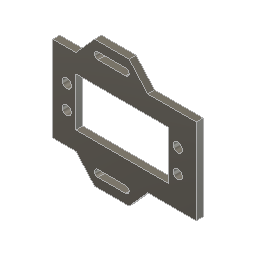
SteeringServoPlatform (Autodesk Fusion 360 design; units mm, degrees)
Autodesk Fusion 360 part; units mm, degrees
sketch "Sketch1" plane through (0, 0, 0) normal (0, 0, 1) x (1, 0, 0)
  line L0 (33.7043, 31.4724) -> (95.7043, 31.4724)
  line L1 (95.7043, 31.4724) -> (95.7043, -5.5276)
  line L2 (95.7043, -5.5276) -> (33.7043, -5.5276)
  line L3 (33.7043, -5.5276) -> (33.7043, 31.4724)
  line L4 (33.7043, 31.4724) -> (43.7043, 31.4724)
  line L5 (43.7043, 31.4724) -> (43.7043, -5.5276)
  line L6 (43.7043, -5.5276) -> (33.7043, -5.5276)
  line L7 (33.7043, -5.5276) -> (33.7043, 31.4724)
  line L8 (95.7043, 31.4724) -> (83.7043, 31.4724)
  line L9 (83.7043, 31.4724) -> (83.7043, -5.5276)
  line L10 (83.7043, -5.5276) -> (95.7043, -5.5276)
  line L11 (95.7043, -5.5276) -> (95.7043, 31.4724)
  line L12 (33.7043, -5.5276) -> (95.7282, -5.5276)
  line L13 (95.7282, -5.5276) -> (95.7282, 2.4724)
  line L14 (95.7282, 2.4724) -> (33.7043, 2.4724)
  line L15 (33.7043, 2.4724) -> (33.7043, -5.5276)
  line L16 (33.7043, 31.4724) -> (95.7282, 31.4724)
  line L17 (95.7282, 31.4724) -> (95.7282, 23.4724)
  line L18 (95.7282, 23.4724) -> (33.7043, 23.4724)
  line L19 (33.7043, 23.4724) -> (33.7043, 31.4724)
  line L20 (33.7043, 2.4724) -> (95.7282, 2.4724)
  line L21 (95.7282, 2.4724) -> (95.7282, -14.5276)
  line L22 (95.7282, -14.5276) -> (33.7043, -14.5276)
  line L23 (33.7043, -14.5276) -> (33.7043, 2.4724)
  line L24 (33.7043, 23.4724) -> (95.7282, 23.4724)
  line L25 (95.7282, 23.4724) -> (95.7282, 40.4724)
  line L26 (95.7282, 40.4724) -> (33.7043, 40.4724)
  line L27 (33.7043, 40.4724) -> (33.7043, 23.4724)
  line L28 (33.7043, -14.5276) -> (95.7282, -14.5276)
  line L29 (95.7282, -14.5276) -> (95.7282, -10.5276)
  line L30 (95.7282, -10.5276) -> (33.7043, -10.5276)
  line L31 (33.7043, -10.5276) -> (33.7043, -14.5276)
  line L32 (33.7043, 40.4724) -> (95.7282, 40.4724)
  line L33 (95.7282, 40.4724) -> (95.7282, 36.4724)
  line L34 (95.7282, 36.4724) -> (33.7043, 36.4724)
  line L35 (33.7043, 36.4724) -> (33.7043, 40.4724)
  line L36 (33.7043, 36.4724) -> (51.7043, 36.4724)
  line L37 (51.7043, 36.4724) -> (51.7043, 31.4724)
  line L38 (51.7043, 31.4724) -> (33.7043, 31.4724)
  line L39 (33.7043, 31.4724) -> (33.7043, 36.4724)
  line L40 (33.7043, -5.5276) -> (51.7043, -5.5276)
  line L41 (51.7043, -5.5276) -> (51.7043, -10.5276)
  line L42 (51.7043, -10.5276) -> (33.7043, -10.5276)
  line L43 (33.7043, -10.5276) -> (33.7043, -5.5276)
  line L44 (51.7043, 36.4724) -> (66.7043, 36.4724)
  line L45 (66.7043, 36.4724) -> (66.7043, 31.4724)
  line L46 (66.7043, 31.4724) -> (51.7043, 31.4724)
  line L47 (51.7043, 31.4724) -> (51.7043, 36.4724)
  line L48 (51.7043, -5.5276) -> (66.7043, -5.5276)
  line L49 (66.7043, -5.5276) -> (66.7043, -10.5276)
  line L50 (66.7043, -10.5276) -> (51.7043, -10.5276)
  line L51 (51.7043, -10.5276) -> (51.7043, -5.5276)
  line L52 (33.7043, -5.5276) -> (95.7282, -5.5276)
  line L53 (95.7282, -5.5276) -> (95.7282, -7.5276)
  line L54 (95.7282, -7.5276) -> (33.7043, -7.5276)
  line L55 (33.7043, -7.5276) -> (33.7043, -5.5276)
  line L56 (33.7043, 31.4724) -> (95.7282, 31.4724)
  line L57 (95.7282, 31.4724) -> (95.7282, 33.4724)
  line L58 (95.7282, 33.4724) -> (33.7043, 33.4724)
  line L59 (33.7043, 33.4724) -> (33.7043, 31.4724)
  line L60 (51.7043, -10.5276) -> (51.7043, -14.5276)
  line L61 (66.7043, -10.5276) -> (66.7043, -14.5276)
  line L62 (51.7043, 36.4724) -> (51.7043, 40.4724)
  line L63 (66.7043, 36.4724) -> (66.7043, 40.4724)
  line L64 (43.7043, 31.4724) -> (51.7043, 40.4724)
  line L65 (43.7043, -5.5276) -> (51.7043, -14.5276)
  line L66 (66.7043, 31.4724) -> (74.7043, 31.4724)
  line L67 (74.7043, 31.4724) -> (74.7043, 40.4724)
  line L68 (74.7043, 40.4724) -> (66.7043, 40.4724)
  line L69 (66.7043, 40.4724) -> (66.7043, 31.4724)
  line L70 (66.7043, 40.4724) -> (74.7043, 31.4724)
  line L71 (66.7043, -5.5276) -> (74.7043, -5.5276)
  line L72 (74.7043, -5.5276) -> (74.7043, -14.5276)
  line L73 (74.7043, -14.5276) -> (66.7043, -14.5276)
  line L74 (66.7043, -14.5276) -> (66.7043, -5.5276)
  line L75 (66.7043, -14.5276) -> (74.7043, -5.5276)
  line L76 (43.7043, 12.9724) -> (41.7043, 12.9724)
  line L77 (41.7043, 12.9724) -> (41.7043, 7.9724)
  line L78 (41.7043, 7.9724) -> (43.7043, 7.9724)
  line L79 (43.7043, 7.9724) -> (43.7043, 12.9724)
  line L80 (43.7043, 12.9724) -> (41.7043, 12.9724)
  line L81 (41.7043, 12.9724) -> (41.7043, 17.9724)
  line L82 (41.7043, 17.9724) -> (43.7043, 17.9724)
  line L83 (43.7043, 17.9724) -> (43.7043, 12.9724)
  line L84 (41.7043, 7.9697) -> (41.7043, 17.9724)
  line L85 (41.7043, 17.9724) -> (37.7043, 17.9724)
  line L86 (37.7043, 17.9724) -> (37.7043, 7.9724)
  line L87 (37.7043, 7.9724) -> (41.7043, 7.9724)
  line L88 (41.7043, 7.9724) -> (41.7043, 17.9724)
  circle A0 centre (39.7043, 17.9724) radius 2
  circle A1 centre (39.7043, 7.9724) radius 2
  line L89 (43.7043, 17.9724) -> (43.7043, 12.9724)
  line L90 (41.7043, 7.9724) -> (41.7043, 17.9724)
  line L91 (41.7043, 12.9724) -> (41.7043, 17.9724)
  line L92 (37.7043, 17.9724) -> (37.7043, 7.9724)
  line L93 (43.7043, 7.9724) -> (43.7043, 12.9724)
  line L94 (41.7043, 7.9697) -> (41.7043, 17.9724)
  circle A2 centre (39.7043, 7.9724) radius 2
  line L95 (43.7043, 12.9724) -> (41.7043, 12.9724)
  line L96 (41.7043, 12.9724) -> (41.7043, 7.9724)
  line L97 (41.7043, 17.9724) -> (37.7043, 17.9724)
  line L98 (41.7043, 7.9724) -> (43.7043, 7.9724)
  circle A3 centre (39.7043, 17.9724) radius 2
  line L99 (43.7043, 12.9724) -> (41.7043, 12.9724)
  line L100 (37.7043, 7.9724) -> (41.7043, 7.9724)
  line L101 (41.7043, 17.9724) -> (43.7043, 17.9724)
  line L102 (41.7043, 7.9697) -> (41.7043, 17.9724)
  line L103 (43.7043, 12.9724) -> (41.7043, 12.9724)
  line L104 (41.7043, 17.9724) -> (43.7043, 17.9724)
  line L105 (41.7043, 17.9724) -> (37.7043, 17.9724)
  line L106 (41.7043, 17.9724) -> (37.7043, 17.9724)
  circle A4 centre (39.7043, 17.9724) radius 2
  circle A5 centre (39.7043, 7.9724) radius 2
  line L107 (43.7043, 7.9724) -> (43.7043, 12.9724)
  line L108 (43.7043, 12.9724) -> (41.7043, 12.9724)
  line L109 (41.7043, 7.9697) -> (41.7043, 17.9724)
  circle A6 centre (39.7043, 17.9724) radius 2
  line L110 (43.7043, 12.9724) -> (41.7043, 12.9724)
  line L111 (37.7043, 7.9724) -> (41.7043, 7.9724)
  line L112 (41.7043, 7.9724) -> (43.7043, 7.9724)
  line L113 (41.7043, 17.9724) -> (43.7043, 17.9724)
  line L114 (41.7043, 7.9724) -> (41.7043, 17.9724)
  line L115 (37.7043, 17.9724) -> (37.7043, 7.9724)
  circle A7 centre (39.7043, 7.9724) radius 2
  line L116 (37.7043, 7.9724) -> (41.7043, 7.9724)
  line L117 (41.7043, 12.9724) -> (41.7043, 7.9724)
  line L118 (43.7043, 7.9724) -> (43.7043, 12.9724)
  line L119 (37.7043, 17.9724) -> (37.7043, 7.9724)
  line L120 (41.7043, 12.9724) -> (41.7043, 17.9724)
  line L121 (43.7043, 12.9724) -> (41.7043, 12.9724)
  line L122 (41.7043, 7.9724) -> (41.7043, 17.9724)
  line L123 (43.7043, 17.9724) -> (43.7043, 12.9724)
  line L124 (43.7043, 17.9724) -> (43.7043, 12.9724)
  line L125 (41.7043, 7.9724) -> (43.7043, 7.9724)
  line L126 (41.7043, 12.9724) -> (41.7043, 7.9724)
  line L127 (41.7043, 12.9724) -> (41.7043, 17.9724)
  line L128 (85.7043, 7.9724) -> (85.7043, 17.9724)
  line L129 (85.7043, 12.9724) -> (85.7043, 17.9724)
  line L130 (85.7043, 7.9697) -> (85.7043, 17.9724)
  line L131 (89.7043, 17.9724) -> (89.7043, 7.9724)
  line L132 (89.7043, 17.9724) -> (89.7043, 7.9724)
  line L133 (83.7043, 17.9724) -> (83.7043, 12.9724)
  line L134 (85.7043, 17.9724) -> (89.7043, 17.9724)
  line L135 (83.7043, 12.9724) -> (85.7043, 12.9724)
  line L136 (85.7043, 12.9724) -> (85.7043, 7.9724)
  line L137 (85.7043, 17.9724) -> (83.7043, 17.9724)
  line L138 (89.7043, 7.9724) -> (85.7043, 7.9724)
  circle A8 centre (87.7043, 17.9724) radius 2
  line L139 (83.7043, 12.9724) -> (85.7043, 12.9724)
  line L140 (85.7043, 7.9724) -> (83.7043, 7.9724)
  line L141 (83.7043, 12.9724) -> (85.7043, 12.9724)
  circle A9 centre (87.7043, 17.9724) radius 2
  line L142 (85.7043, 7.9724) -> (83.7043, 7.9724)
  line L143 (83.7043, 7.9724) -> (83.7043, 12.9724)
  circle A10 centre (87.7043, 7.9724) radius 2
  line L144 (85.7043, 7.9724) -> (83.7043, 7.9724)
  circle A11 centre (87.7043, 17.9724) radius 2
  line L145 (83.7043, 12.9724) -> (85.7043, 12.9724)
  line L146 (85.7043, 17.9724) -> (89.7043, 17.9724)
  line L147 (83.7043, 12.9724) -> (85.7043, 12.9724)
  circle A12 centre (87.7043, 17.9724) radius 2
  line L148 (85.7043, 17.9724) -> (83.7043, 17.9724)
  line L149 (85.7043, 17.9724) -> (83.7043, 17.9724)
  line L150 (85.7043, 17.9724) -> (89.7043, 17.9724)
  line L151 (85.7043, 17.9724) -> (83.7043, 17.9724)
  line L152 (85.7043, 17.9724) -> (89.7043, 17.9724)
  circle A13 centre (87.7043, 7.9724) radius 2
  line L153 (89.7043, 7.9724) -> (85.7043, 7.9724)
  line L154 (85.7043, 12.9724) -> (85.7043, 17.9724)
  line L155 (89.7043, 7.9724) -> (85.7043, 7.9724)
  line L156 (85.7043, 12.9724) -> (85.7043, 17.9724)
  line L157 (83.7043, 7.9724) -> (83.7043, 12.9724)
  line L158 (89.7043, 7.9724) -> (85.7043, 7.9724)
  circle A14 centre (87.7043, 7.9724) radius 2
  line L159 (83.7043, 17.9724) -> (83.7043, 12.9724)
  line L160 (85.7043, 7.9724) -> (85.7043, 17.9724)
  line L161 (85.7043, 12.9724) -> (85.7043, 17.9724)
  line L162 (85.7043, 7.9697) -> (85.7043, 17.9724)
  line L163 (89.7043, 17.9724) -> (89.7043, 7.9724)
  line L164 (85.7043, 7.9724) -> (85.7043, 17.9724)
  line L165 (89.7043, 17.9724) -> (89.7043, 7.9724)
  line L166 (85.7043, 7.9724) -> (85.7043, 17.9724)
  line L167 (83.7043, 17.9724) -> (83.7043, 12.9724)
  line L168 (85.7043, 7.9724) -> (83.7043, 7.9724)
  line L169 (83.7043, 12.9724) -> (85.7043, 12.9724)
  line L170 (85.7043, 12.9724) -> (85.7043, 7.9724)
  line L171 (85.7043, 12.9724) -> (85.7043, 7.9724)
  line L172 (85.7043, 12.9724) -> (85.7043, 7.9724)
  line L173 (85.7043, 7.9697) -> (85.7043, 17.9724)
  line L174 (83.7043, 17.9724) -> (83.7043, 12.9724)
  line L175 (85.7043, 7.9697) -> (85.7043, 17.9724)
  line L176 (83.7043, 7.9724) -> (83.7043, 12.9724)
  line L177 (83.7043, 12.9724) -> (85.7043, 12.9724)
  line L178 (83.7043, 12.9724) -> (85.7043, 12.9724)
  line L179 (83.7043, 7.9724) -> (83.7043, 12.9724)
  circle A15 centre (87.7043, 7.9724) radius 2
  circle A16 centre (65.2043, 34.9724) radius 1.5
  circle A17 centre (53.2043, 34.9724) radius 1.5
  circle A18 centre (53.2043, -9.0276) radius 1.5
  circle A19 centre (65.2043, -9.0276) radius 1.5
  dimension "d1" = 62
  dimension "d2" = 37
  dimension "d3" = 10
  dimension "d4" = 12
  dimension "d5" = 8
  dimension "d6" = 8
  dimension "d7" = 17
  dimension "d8" = 17
  dimension "d9" = 4
  dimension "d10" = 4
  dimension "d11" = 18
  dimension "d12" = 18
  dimension "d13" = 15
  dimension "d14" = 15
  dimension "d15" = 2
  dimension "d16" = 2
  dimension "d17" = 4
  dimension "d18" = 4
  dimension "d19" = 4
  dimension "d20" = 4
  dimension "d21" = 8
  dimension "d22" = 8
  dimension "d23" = 2
  dimension "d24" = 5
  dimension "d25" = 2
  dimension "d26" = 5
  dimension "d30" = 4
  dimension "d31" = 4
  dimension "d32" = 4
  dimension "d33" = 2
  dimension "d34" = 5
  dimension "d35" = 2
  dimension "d36" = 5
  dimension "d37" = 4
  dimension "d38" = 4
  dimension "d39" = 4
  dimension "d40" = 2
  dimension "d41" = 5
  dimension "d42" = 2
  dimension "d43" = 5
  dimension "d44" = 4
  dimension "d45" = 4
  dimension "d46" = 4
  dimension "d47" = 2
  dimension "d48" = 5
  dimension "d49" = 2
  dimension "d50" = 5
  dimension "d51" = 4
  dimension "d52" = 4
  dimension "d53" = 4
  dimension "d54" = 2
  dimension "d55" = 5
  dimension "d56" = 2
  dimension "d57" = 5
  dimension "d58" = 4
  dimension "d59" = 4
  dimension "d60" = 4
  dimension "d61" = 2
  dimension "d62" = 5
  dimension "d63" = 2
  dimension "d64" = 5
  dimension "d65" = 4
  dimension "d66" = 4
  dimension "d67" = 4
  dimension "d68" = 2
  dimension "d69" = 5
  dimension "d70" = 2
  dimension "d71" = 5
  dimension "d72" = 4
  dimension "d73" = 4
  dimension "d74" = 4
  dimension "d75" = 2
  dimension "d76" = 5
  dimension "d77" = 2
  dimension "d78" = 5
  dimension "d79" = 4
  dimension "d80" = 4
  dimension "d81" = 4
  dimension "d82" = 3
  dimension "d83" = 3
  dimension "d84" = 3
  dimension "d85" = 3
  constraint horizontal L0
  constraint vertical L1
  constraint horizontal L2
  constraint vertical L3
  constraint horizontal L4
  constraint vertical L5
  constraint horizontal L6
  constraint vertical L7
  constraint horizontal L8
  constraint vertical L9
  constraint horizontal L10
  constraint vertical L11
  constraint horizontal L12
  constraint vertical L13
  constraint horizontal L14
  constraint vertical L15
  constraint horizontal L16
  constraint vertical L17
  constraint horizontal L18
  constraint vertical L19
  constraint horizontal L20
  constraint vertical L21
  constraint horizontal L22
  constraint vertical L23
  constraint horizontal L24
  constraint vertical L25
  constraint horizontal L26
  constraint vertical L27
  constraint horizontal L28
  constraint vertical L29
  constraint horizontal L30
  constraint vertical L31
  constraint horizontal L32
  constraint vertical L33
  constraint horizontal L34
  constraint vertical L35
  constraint horizontal L36
  constraint vertical L37
  constraint horizontal L38
  constraint vertical L39
  constraint horizontal L40
  constraint vertical L41
  constraint horizontal L42
  constraint vertical L43
  constraint horizontal L44
  constraint vertical L45
  constraint horizontal L46
  constraint vertical L47
  constraint horizontal L48
  constraint vertical L49
  constraint horizontal L50
  constraint vertical L51
  constraint horizontal L52
  constraint vertical L53
  constraint horizontal L54
  constraint vertical L55
  constraint horizontal L56
  constraint vertical L57
  constraint horizontal L58
  constraint vertical L59
  constraint perpendicular L22 L60
  constraint perpendicular L22 L61
  constraint perpendicular L44 L62
  constraint perpendicular L34 L63
  constraint horizontal L66
  constraint vertical L67
  constraint horizontal L68
  constraint vertical L69
  constraint horizontal L71
  constraint vertical L72
  constraint horizontal L73
  constraint vertical L74
  constraint horizontal L76
  constraint vertical L77
  constraint horizontal L78
  constraint vertical L79
  constraint midpoint L5 L76.start
  constraint horizontal L80
  constraint vertical L81
  constraint horizontal L82
  constraint vertical L83
  constraint vertical L84
  constraint horizontal L85
  constraint vertical L86
  constraint horizontal L87
  constraint vertical L88
  constraint midpoint L85 A0.centre
  constraint midpoint L87 A1.centre
  constraint horizontal L95
  constraint vertical L96
  constraint horizontal L98
  constraint vertical L93
  constraint horizontal L99
  constraint vertical L91
  constraint horizontal L101
  constraint vertical L89
  constraint vertical L94
  constraint horizontal L97
  constraint vertical L92
  constraint horizontal L100
  constraint vertical L90
  constraint midpoint A0.centre L97
  constraint midpoint A1.centre L100
  constraint horizontal L121
  constraint vertical L117
  constraint horizontal L112
  constraint vertical L118
  constraint horizontal L110
  constraint vertical L127
  constraint horizontal L113
  constraint vertical L123
  constraint vertical L109
  constraint horizontal L106
  constraint vertical L115
  constraint horizontal L116
  constraint vertical L122
  constraint midpoint A0.centre L106
  constraint midpoint A1.centre L116
  constraint horizontal L103
  constraint vertical L126
  constraint horizontal L125
  constraint vertical L107
  constraint horizontal L108
  constraint vertical L120
  constraint horizontal L104
  constraint vertical L124
  constraint vertical L102
  constraint horizontal L105
  constraint vertical L119
  constraint horizontal L111
  constraint vertical L114
  constraint midpoint A0.centre L105
  constraint midpoint A1.centre L111
  constraint midpoint A8.centre L150
  constraint midpoint A10.centre L138
  constraint midpoint A8.centre L146
  constraint midpoint A10.centre L153
  constraint midpoint A8.centre L134
  constraint midpoint A10.centre L158
  constraint midpoint A8.centre L152
  constraint midpoint A10.centre L155
  constraint tangent L69 A16
  constraint tangent L34 A16
  constraint tangent L47 A17
  constraint tangent L44 A17
  constraint tangent L41 A18
  constraint tangent L54 A18
  constraint tangent L74 A19
  constraint tangent L50 A19
  measures "d1" distance of L0.start L0.end
  measures "d2" distance of L0.start L2.end
  measures "d3" distance of L0.start L4.end
  measures "d4" distance of L0.end L8.end
  measures "d5" distance of L2.end L14.end
  measures "d6" distance of L0.start L18.end
  measures "d7" distance of L14.end L22.end
  measures "d8" distance of L18.end L26.end
  measures "d9" distance of L22.end L30.end
  measures "d10" distance of L26.end L34.end
  measures "d11" distance of L34.end L36.end
  measures "d12" distance of L2.end L40.end
  measures "d13" distance of L36.end L44.end
  measures "d14" distance of L40.end L48.end
  measures "d15" distance of L2.end L54.end
  measures "d16" distance of L0.start L58.end
  measures "d17" distance of L41.end L60.end
  measures "d18" distance of L49.end L61.end
  measures "d19" distance of L36.end L62.end
  measures "d20" distance of L44.end L63.end
  measures "d21" distance of L45.end L66.end
  measures "d22" distance of L48.end L71.end
  measures "d23" distance of L76.start L76.end
  measures "d24" distance of L76.start L78.end
  measures "d25" distance of L76.start L76.end
  measures "d26" distance of L76.start L82.end
  measures "d30" distance of L81.end L85.end
  measures "d31" diameter of A0
  measures "d32" diameter of A1
  measures "d33" distance of L76.start L76.end
  measures "d34" distance of L78.end L76.start
  measures "d35" distance of L76.start L76.end
  measures "d36" distance of L76.start L82.end
  measures "d37" distance of L81.end L85.end
  measures "d38" diameter of A3
  measures "d39" diameter of A2
  measures "d40" distance of L76.start L76.end
  measures "d41" distance of L78.end L76.start
  measures "d42" distance of L76.start L76.end
  measures "d43" distance of L76.start L82.end
  measures "d44" distance of L81.end L85.end
  measures "d45" diameter of A4
  measures "d46" diameter of A5
  measures "d47" distance of L76.start L76.end
  measures "d48" distance of L78.end L76.start
  measures "d49" distance of L76.start L76.end
  measures "d50" distance of L76.start L82.end
  measures "d51" distance of L85.end L81.end
  measures "d52" diameter of A6
  measures "d53" diameter of A7
  measures "d54" distance of L133.end L129.start
  measures "d55" distance of L140.end L133.end
  measures "d56" distance of L133.end L129.start
  measures "d57" distance of L133.end L133.start
  measures "d58" distance of L128.end L131.start
  measures "d59" diameter of A11
  measures "d60" diameter of A14
  measures "d61" distance of L133.end L129.start
  measures "d62" distance of L140.end L133.end
  measures "d63" distance of L133.end L129.start
  measures "d64" distance of L133.end L133.start
  measures "d65" distance of L131.start L128.end
  measures "d66" diameter of A8
  measures "d67" diameter of A13
  measures "d68" distance of L133.end L129.start
  measures "d69" distance of L140.end L133.end
  measures "d70" distance of L129.start L133.end
  measures "d71" distance of L133.start L133.end
  measures "d72" distance of L131.start L128.end
  measures "d73" diameter of A9
  measures "d74" diameter of A15
  measures "d75" distance of L133.end L129.start
  measures "d76" distance of L133.end L140.end
  measures "d77" distance of L129.start L133.end
  measures "d78" distance of L133.start L133.end
  measures "d79" distance of L131.start L128.end
  measures "d80" diameter of A12
  measures "d81" diameter of A10
  measures "d82" diameter of A16
  measures "d83" diameter of A17
  measures "d84" diameter of A18
  measures "d85" diameter of A19
extrude "Extrude1" add sketch "Sketch1" along normal blind 3 contours L0 L3 L4 L5 L7 L16 L18 L19 L24 L27 L38 L56 | L0 L16 L37 L38 L47 L56 L58 L64 | L0 L5 L9 L16 L18 L24 L38 L46 L56 L66 | L3 L5 L7 L14 L18 L20 L24 L78 L82 L84 L86 A0 A1 L92 L94 A2 L98 A3 L101 L102 L104 A4 A5 L109 A6 L112 L113 L115 A7 L119 L125 | L0 L16 L37 L45 L46 L47 L56 L58 L69 | L34 L36 L37 L47 L58 L64 | L2 L3 L5 L6 L7 L12 L14 L15 L20 L23 L40 L52 | L0 L16 L45 L56 L58 L66 L69 L70 | L37 L47 L58 A17 | L5 L76 L80 L81 L82 L83 L84 L88 L89 L90 L91 L94 L95 L99 L101 L102 L103 L104 L108 L109 L110 L113 L114 L120 L121 L122 L123 L124 L127 | L1 L9 L11 L14 L18 L20 L24 L130 L131 L132 L137 A8 L140 A9 L142 A10 L144 A11 A12 L148 L149 L151 A13 A14 L162 L163 L165 L168 L173 L175 A15 | L0 L1 L8 L9 L11 L16 L18 L24 L56 | L34 L36 L62 L64 | L2 L5 L9 L12 L14 L20 L40 L48 L52 L71 | L45 L58 L69 A16 | L34 L45 L58 L69 L70 | L34 L37 L44 L47 A17 | L5 L76 L77 L78 L79 L80 L84 L88 L90 L93 L94 L95 L96 L98 L99 L102 L103 L107 L108 L109 L110 L112 L114 L117 L118 L121 L122 L125 L126 | L77 L81 L84 L86 L88 A0 A1 L90 L91 L92 L94 A2 L96 A3 L102 A4 A5 L109 A6 L114 L115 A7 L117 L119 L120 L122 L126 L127 | L9 L128 L129 L130 L133 L135 L137 L139 L141 L145 L147 L148 L149 L151 L154 L156 L159 L160 L161 L162 L164 L166 L167 L169 L173 L174 L175 L177 L178 | L26 L32 L34 L44 L62 L63 L69 | L2 L12 L40 L41 L51 L52 L54 L65 | L1 L2 L9 L10 L11 L12 L14 L20 L52 | L34 L44 L45 L69 A16 | L9 L128 L130 L135 L136 L139 L140 L141 L142 L143 L144 L145 L147 L157 L160 L162 L164 L166 L168 L169 L170 L171 L172 L173 L175 L176 L177 L178 L179 | L128 L129 L130 L131 L132 L136 A8 A9 A10 A11 A12 A13 L154 L156 A14 L160 L161 L162 L163 L164 L165 L166 L170 L171 L172 L173 L175 A15 | L34 L63 L69 L70 | L2 L12 L41 L48 L49 L51 L52 L54 L74 | L30 L41 L42 L51 L54 L65 | L2 L12 L49 L52 L54 L71 L74 L75 | L41 L51 L54 A18 | L30 L42 L60 L65 | L30 L49 L54 L74 L75 | L49 L54 L74 A19 | L30 L41 L50 L51 A18 | L22 L28 L30 L50 L60 L61 L74 | L30 L49 L50 L74 A19 | L30 L61 L74 L75
